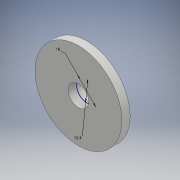
# Autodesk Inventor part: maingear
Saved by Autodesk Inventor 2018.3 (Build 223284000, 284)
## iProperties
Created: 2019-10-08
Part Number: maingear
Material: 一般
Document SubType Name: Modeling
Designer: Eiji Nishizawa
Density: 1 g/cm^3
Appearance: 既定
Author: Eiji Nishizawa
Autodesk Inventor part; units mm, degrees
ref_plane "YZ Plane" through (0, 0, 0) normal (1, 0, 0) x (0, 1, 0)
ref_plane "XZ Plane" through (0, 0, 0) normal (0, 1, 0) x (-1, 0, 0)
ref_plane "XY Plane" through (0, 0, 0) normal (0, 0, 1) x (1, 0, 0)
sketch "スケッチ1" plane through (0, 0, 0) normal (0, 1, 0) x (-1, 0, 0)
  circle A0 centre (0, 0) radius 28
  circle A1 centre (0, 0) radius 26.2665
  dimension "d0" = 56
  constraints: 2 centre point, 2 coincident
  measures "d0" diameter of A0
extrude "押し出し1" add sketch "スケッチ1" along normal blind 5 contours A1
sketch "スケッチ2" plane through (0, 5, 0) normal (0, 1, 0) x (1, 0, 0)
  circle A0 centre (0, 0) radius 6.2
  circle A1 centre (0, 0) radius 8
  dimension "d3" = 16
  dimension "d9" = 12.4
  constraints: 2 centre point, 2 coincident
  measures "d3" diameter of A1
  measures "d9" diameter of A0
extrude "押し出し2" cut sketch "スケッチ2" against normal blind 5 contours A0
extrude "押し出し3" add sketch "スケッチ2" along normal blind 9
